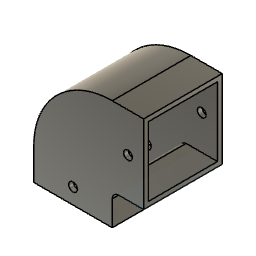
Elbow v2 (Autodesk Fusion 360 design; units mm, degrees)
Autodesk Fusion 360 part; units mm, degrees
note: some values were not read from the file. Set by a fixed rule: which sketch regions a step uses.
sketch "Sketch1" plane through (0, 0, 0) normal (0, 0, 1) x (1, 0, 0)
  line L0 (13.97, 13.97) -> (-13.97, 13.97)
  line L1 (-13.97, 13.97) -> (-13.97, -13.97)
  line L2 (-13.97, -13.97) -> (13.97, -13.97)
  line L3 (13.97, -13.97) -> (13.97, 13.97)
  line L4 (13.97, 13.97) -> (-13.97, -13.97) construction
  line L5 (-13.97, 13.97) -> (13.97, -13.97) construction
  line L6 (15.875, 15.875) -> (-15.875, 15.875)
  line L7 (-15.875, 15.875) -> (-15.875, -15.875)
  line L8 (-15.875, -15.875) -> (15.875, -15.875)
  line L9 (15.875, -15.875) -> (15.875, 15.875)
  line L10 (15.875, 15.875) -> (-15.875, -15.875) construction
  line L11 (-15.875, 15.875) -> (15.875, -15.875) construction
  dimension "d1" = 27.94
  dimension "d2" = 27.94
  dimension "d3" = 31.75
  dimension "d4" = 31.75
  constraint horizontal L0
  constraint perpendicular L0 L1
  constraint parallel L0 L2
  constraint parallel L1 L3
  constraint coincident L4 origin
  constraint coincident L5 origin
  constraint horizontal L6
  constraint perpendicular L6 L7
  constraint parallel L6 L8
  constraint parallel L7 L9
  constraint coincident L10 origin
  constraint coincident L11 origin
  measures "d1" distance of L1.end L2.end
  measures "d2" distance of L0.end L1.end
  measures "d3" distance of L7.end L8.end
  measures "d4" distance of L6.start L8.end
extrude "Extrude1" add sketch "Sketch1" along normal blind 12.7
revolve "Revolve1" add 1 faces at (-15.24, -4.6567, 12.7) angle 90 about axis through (15.875, -15.875, 12.7) along (0, 1, 0)
sketch "Sketch3" plane through (15.875, 0, 0) normal (1, 0, 0) x (0, 1, 0)
  line L0 (13.97, 14.605) -> (-13.97, 14.605)
  line L1 (-13.97, 14.605) -> (-13.97, 42.545)
  line L2 (-13.97, 42.545) -> (13.97, 42.545)
  line L3 (13.97, 42.545) -> (13.97, 14.605)
  line L4 (-15.875, 0) -> (15.875, 0)
  line L5 (15.875, 0) -> (15.875, 44.45)
  line L6 (15.875, 44.45) -> (-15.875, 44.45)
  line L7 (-15.875, 44.45) -> (-15.875, 0)
  line L8 (-13.97, 42.545) -> (13.97, 42.545)
  line L9 (13.97, 42.545) -> (13.97, 14.605)
  line L10 (13.97, 14.605) -> (-13.97, 14.605)
  line L11 (-13.97, 14.605) -> (-13.97, 42.545)
  line L12 (-15.875, 44.45) -> (14.2875, 44.45)
  line L13 (14.2875, 12.7) -> (-15.875, 12.7)
  line L14 (-15.875, 12.7) -> (-15.875, 44.45)
  line L15 (14.2875, 12.7) -> (15.875, 12.7)
  dimension "d10" = 31.75
  constraint horizontal L8
  constraint vertical L9
  constraint horizontal L10
  constraint vertical L11
  constraint coincident L0.start L3.end
  constraint coincident L1.end L2.start
  constraint horizontal L12
  constraint horizontal L13
  constraint vertical L14
  constraint coincident L6.end L7.start
  constraint coincident L5 L15.end
  constraint perpendicular L5 L15
  measures "d10" distance of L6.end L13.end
extrude "Extrude2" add sketch "Sketch3" along normal blind 12.7 contours L5 L6 L7 L12 L13 L14 L15
fillet "Fillet1" radius 2.54 1 edges at (15.875, 0, 12.7)
sketch "Sketch5" plane through (0, 0, 12.7) normal (0, 0, -1) x (1, 0, 0)
  line L0 (18.415, 15.875) -> (18.415, -15.875)
  line L1 (18.415, -15.875) -> (28.575, -15.875)
  line L2 (28.575, -15.875) -> (28.575, 15.875)
  line L3 (28.575, 15.875) -> (18.415, 15.875)
sketch "Sketch6" plane through (0, -15.875, 0) normal (0, -1, 0) x (1, 0, 0)
  line L0 (-15.875, 0) -> (15.875, 0)
  line L1 (15.875, 0) -> (15.875, 10.16)
  arc A0 (18.415, 12.7) -> (15.875, 10.16) centre (18.415, 10.16) ccw
  line L2 (18.415, 12.7) -> (28.575, 12.7)
  line L3 (28.575, 12.7) -> (28.575, 44.45)
  line L4 (28.575, 44.45) -> (15.875, 44.45)
  arc A1 (15.875, 44.45) -> (-15.875, 12.7) centre (15.875, 12.7) ccw
  line L5 (-15.875, 12.7) -> (-15.875, 0)
  circle A2 centre (22.225, 28.575) radius 1.778
  line L6 (28.575, 12.7) -> (18.415, 12.7)
  dimension "d19" = 3.556
  dimension "d20" = 6.35
  dimension "d21" = 15.875
  measures "d19" diameter of A2
  measures "d20" distance of L3 A2.centre
  measures "d21" distance of A2.centre L6
extrude "Extrude4" cut sketch "Sketch6" against normal blind 33.02 contours A2
sketch "Sketch7" plane through (0, -15.875, 0) normal (0, -1, 0) x (1, 0, 0)
  circle A0 centre (22.225, 28.575) radius 1.778
  line L0 (-15.875, 0) -> (15.875, 0)
  line L1 (15.875, 0) -> (15.875, 10.16)
  arc A1 (18.415, 12.7) -> (15.875, 10.16) centre (18.415, 10.16) ccw
  line L2 (18.415, 12.7) -> (28.575, 12.7)
  line L3 (28.575, 12.7) -> (28.575, 44.45)
  line L4 (28.575, 44.45) -> (15.875, 44.45)
  arc A2 (15.875, 44.45) -> (-15.875, 12.7) centre (15.875, 12.7) ccw
  line L5 (-15.875, 12.7) -> (-15.875, 0)
  circle A3 centre (0, 6.35) radius 1.778
  dimension "d24" = 3.556
  dimension "d25" = 6.35
  dimension "d26" = 15.875
  measures "d24" diameter of A3
  measures "d25" distance of L0 A3.centre
  measures "d26" distance of L5 A3.centre
extrude "Extrude5" cut sketch "Sketch7" against normal blind 35.56 contours A3
equation "d21 = ( 1.25 / 2 ) * 1 in"
